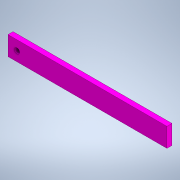
# Autodesk Inventor part: handle
Saved by Autodesk Inventor 2020.3 (Build 243373000, 373)
## iProperties
Created: 2021-06-19
Part Number: handle
Material: Steel, Mild
Document SubType Name: Modeling
Designer: 0x6f736f646f
Density: 7.85 g/cm^3
Appearance: Magenta
Author: 0x6f736f646f
Autodesk Inventor part; units mm, degrees
ref_plane "YZ Plane" through (0, 0, 0) normal (1, 0, 0) x (0, 1, 0)
ref_plane "XZ Plane" through (0, 0, 0) normal (0, 1, 0) x (-1, 0, 0)
ref_plane "XY Plane" through (0, 0, 0) normal (0, 0, 1) x (1, 0, 0)
sketch "Sketch1" plane through (0, 0, 0) normal (0, 0, 1) x (1, 0, 0)
  line L0 (0, 0) -> (-300, 0)
  line L1 (-300, 0) -> (-300, 36)
  line L2 (-300, 36) -> (0, 36)
  line L3 (0, 36) -> (0, 0)
  circle A0 centre (-283, 18) radius 5
  dimension "d0" = 300
  dimension "d1" = 36
  dimension "d2" = 10
  dimension "d3" = 17
  dimension "d4" = 18
  constraints: 8 end point, 2 parallel, 1 centre point, 1 horizontal, 1 perpendicular
  measures "d0" distance of L0.start L0.end
  measures "d1" distance of L2.end L0.start
  measures "d2" diameter of A0
  measures "d3" distance from line of L1 A0.centre
  measures "d4" distance from line of L0 A0.centre
extrude "Extrusion1" add sketch "Sketch1" along normal blind 9.525
body "Solid1"
